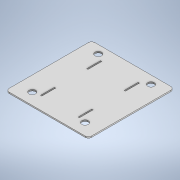
# Autodesk Inventor part: plade_til_beslag
Saved by Autodesk Inventor 2022 (Build 260153000, 153)
## iProperties
Created: 2022-04-09
Part Number: plade_til_beslag
Material: Generic
Document SubType Name: Modeling
Designer: Patrick
Density: 1 g/cm^3
Appearance: Default
Author: Patrick
Autodesk Inventor part; units mm, degrees
ref_plane "YZ Plane" through (0, 0, 0) normal (1, 0, 0) x (0, 1, 0)
ref_plane "XZ Plane" through (0, 0, 0) normal (0, 1, 0) x (-1, 0, 0)
ref_plane "XY Plane" through (0, 0, 0) normal (0, 0, 1) x (1, 0, 0)
sketch "Sketch1" plane through (0, 0, 0) normal (0, 1, 0) x (-1, 0, 0)
  line L0 (0, 0) -> (125, 0)
  line L1 (125, 0) -> (125, -130)
  line L2 (125, -130) -> (0, -130)
  line L3 (0, -130) -> (0, 0)
  circle A0 centre (102.5, -17.5) radius 5
  circle A1 centre (102.5, -117.5) radius 5
  circle A2 centre (22.5, -17.5) radius 5
  circle A3 centre (22.5, -117.5) radius 5
  dimension "d0" = 130
  dimension "d1" = 125
  dimension "d2" = 10
  dimension "d3" = 10
  dimension "d4" = 100
  dimension "d5" = 10
  dimension "d6" = 10
  dimension "d7" = 100
  dimension "d8" = 80
  dimension "d9" = 80
  dimension "d10" = 17.5
  dimension "d11" = 22.5
  dimension "d12" = 17.5
  dimension "d13" = 22.5
  constraints: 8 end point, 4 centre point, 2 parallel, 1 horizontal, 1 perpendicular
  measures "d0" distance of L0.end L1.end
  measures "d1" distance of L1.end L2.end
  measures "d2" diameter of A0
  measures "d3" diameter of A1
  measures "d4" distance of A1.centre A0.centre
  measures "d5" diameter of A2
  measures "d6" diameter of A3
  measures "d7" distance of A3.centre A2.centre
  measures "d8" distance of A2.centre A0.centre
  measures "d9" distance of A3.centre A1.centre
  measures "d10" distance from line of L0 A0.centre
  measures "d11" distance from line of L1 A0.centre
  measures "d12" distance from line of L0 A2.centre
  measures "d13" distance from line of L3 A3.centre
extrude "Extrusion1" add sketch "Sketch1" along normal blind 2
sketch "Sketch2" plane through (0, 2, 0) normal (0, 1, 0) x (1, 0, 0)
  line L0 (-90, 115.6784) -> (-35, 115.6784) construction
  line L1 (-35, 115.6784) -> (-35, 15.6784) construction
  line L2 (-35, 15.6784) -> (-90, 15.6784) construction
  line L3 (-90, 15.6784) -> (-90, 115.6784) construction
  line L4 (0, 130) -> (-125, 130) projected
  line L5 (-125, 130) -> (-125, 0) projected
  line L6 (-125, 0) -> (0, 0) projected
  line L7 (0, 0) -> (0, 130) projected
  circle A0 centre (-22.5, 117.5) radius 5 projected
  circle A1 centre (-22.5, 17.5) radius 5 projected
  circle A2 centre (-102.5, 117.5) radius 5 projected
  circle A3 centre (-102.5, 17.5) radius 5 projected
  line L8 (-35, 40.5) -> (-33, 40.5)
  line L9 (-33, 40.5) -> (-33, 19.5)
  line L10 (-33, 19.5) -> (-35, 19.5)
  line L11 (-35, 19.5) -> (-35, 40.5)
  line L12 (-35, 110.5) -> (-33, 110.5)
  line L13 (-33, 110.5) -> (-33, 89.5)
  line L14 (-33, 89.5) -> (-35, 89.5)
  line L15 (-35, 89.5) -> (-35, 110.5)
  line L16 (-90, 110.5) -> (-92, 110.5)
  line L17 (-92, 110.5) -> (-92, 89.5)
  line L18 (-92, 89.5) -> (-90, 89.5)
  line L19 (-90, 89.5) -> (-90, 110.5)
  line L20 (-90, 40.5) -> (-92, 40.5)
  line L21 (-92, 40.5) -> (-92, 19.5)
  line L22 (-92, 19.5) -> (-90, 19.5)
  line L23 (-90, 19.5) -> (-90, 40.5)
  dimension "d16" = 55
  dimension "d17" = 100
  dimension "d18" = 125
  dimension "d19" = 35
  dimension "d20" = 2
  dimension "d21" = 2
  dimension "d22" = 2
  dimension "d23" = 2
  dimension "d24" = 21
  dimension "d25" = 21
  dimension "d26" = 21
  dimension "d27" = 21
  dimension "d28" = 19.5
  dimension "d29" = 19.5
  dimension "d30" = 19.5
  dimension "d31" = 19.5
  constraints: 40 end point, 10 parallel, 5 horizontal, 5 perpendicular, 5 point on line
  measures "d16" distance between parallel lines of L1 L3
  measures "d17" distance of L0.end L1.end
  measures "d18" distance of L5.end L6.end
  measures "d19" distance between parallel lines of L7 L1
  measures "d20" distance between parallel lines of L3 L17
  measures "d21" distance between parallel lines of L3 L21
  measures "d22" distance between parallel lines of L15 L13
  measures "d23" distance between parallel lines of L1 L9
  measures "d24" distance of L8.end L9.end
  measures "d25" distance of L12.end L13.end
  measures "d26" distance of L20.end L21.end
  measures "d27" distance of L16.end L17.end
  measures "d28" distance between parallel lines of L4 L12
  measures "d29" distance between parallel lines of L6 L10
  measures "d30" distance between parallel lines of L6 L22
  measures "d31" distance between parallel lines of L4 L16
extrude "Extrusion2" cut sketch "Sketch2" against normal through all contours L8 L9 L10 L11 | L12 L13 L14 L15 | L19 L18 L17 L16 | L23 L22 L21 L20
fillet "Fillet1" radius 5 4 edges at (0, 1, 0) (0, 1, -130) (-125, 1, 0) (-125, 1, -130)
equation "\"d19\" = -0.5 * d16 + 0.5 * d18"
equation "\"d25\" = d24"
equation "\"d26\" = d27"
equation "\"d27\" = d25"
equation "\"d29\" = d28"
equation "\"d30\" = d29"
equation "\"d31\" = d28"
body "Solid1"
